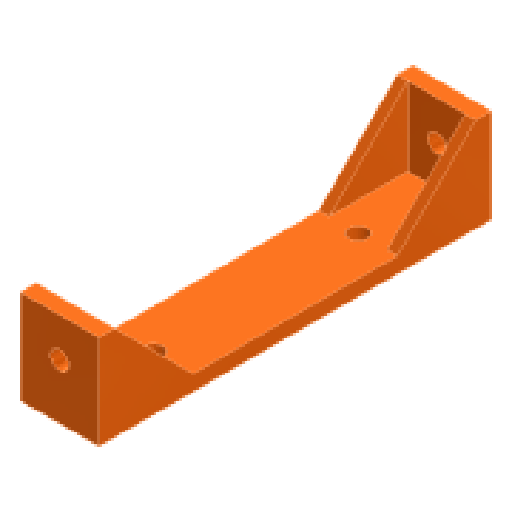
# Autodesk Inventor part: Frame_Brace_Mount
Saved by Autodesk Inventor 2023.2 (Build 272271000, 271)
## iProperties
Created: 2023-02-02
Part Number: Frame_Brace_Mount
Material: ABS Plastic
Document SubType Name: Modeling
Designer: remop
Density: 1.06 g/cm^3
Appearance: Smooth - Light Orange
Author: remop
Autodesk Inventor part; units mm, degrees
ref_plane "YZ Plane" through (0, 0, 0) normal (1, 0, 0) x (0, 1, 0)
ref_plane "XZ Plane" through (0, 0, 0) normal (0, 1, 0) x (-1, 0, 0)
ref_plane "XY Plane" through (0, 0, 0) normal (0, 0, 1) x (1, 0, 0)
sketch "Sketch1" plane through (0, 0, 0) normal (0, 1, 0) x (-1, 0, 0)
  line L0 (-7.5, 37.5) -> (7.5, 37.5)
  line L1 (7.5, 37.5) -> (7.5, -37.5)
  line L2 (7.5, -37.5) -> (-7.5, -37.5)
  line L3 (-7.5, -37.5) -> (-7.5, 37.5)
  line L4 (-7.5, 37.5) -> (7.5, -37.5) construction
  line L5 (7.5, 37.5) -> (-7.5, -37.5) construction
  circle A0 centre (0, 19.5) radius 1.75
  circle A1 centre (0, -19.5) radius 1.75
  point P0 (0, 0)
  point P1 (0, -37.5)
  dimension "d0" = 15
  dimension "d1" = 75
  dimension "d13" = 18
  dimension "d14" = 18
  dimension "d16" = 3.5
  constraints: 12 end point, 3 midpoint, 2 centre point, 2 parallel, 2 vertical alignment, 1 equal radius, 1 horizontal, 1 perpendicular
  measures "d0" distance of L1.end L2.end
  measures "d1" distance of L2.end L0.start
  measures "d13" distance from line of L0 A0.centre
  measures "d14" distance from line of L2 A1.centre
  measures "d16" diameter of A1
extrude "Extrusion1" add sketch "Sketch1" along normal blind 3
sketch "Sketch2" plane through (-7.5, 0, 37.5) normal (0, 0, 1) x (1, 0, 0)
  line L0 (0, 0) -> (15, 0) projected
  line L1 (15, 0) -> (15, 3) projected
  line L2 (0, 3) -> (15, 3) projected
  line L3 (0, 0) -> (0, 3) projected
  line L4 (15, 3) -> (0, 3) projected
  line L5 (0, 3) -> (15, 3)
  line L6 (15, 3) -> (15, 18)
  line L7 (15, 18) -> (0, 18)
  line L8 (0, 18) -> (0, 3)
  circle A0 centre (7.5, 10.5) radius 1.75
  point P0 (7.5, 0)
  point P1 (7.5, 18)
  point P2 (0, 10.5)
  dimension "d15" = 3.5
  constraints: 8 end point, 2 midpoint, 2 parallel, 2 perpendicular, 1 centre point, 1 coincident, 1 horizontal, 1 horizontal alignment, 1 vertical alignment
  measures "d15" diameter of A0
extrude "Extrusion2" add sketch "Sketch2" against normal blind 3 contours L8 L7 L6 L2
sketch "Sketch3" plane through (7.5, 0, -37.5) normal (0, 0, -1) x (-1, 0, 0)
  line L0 (15, 18) -> (0, 18) projected
  line L1 (0, 18) -> (0, 3) projected
  line L2 (15, 3) -> (0, 3) projected
  line L3 (15, 3) -> (15, 18) projected
  circle A0 centre (7.5, 10.5) radius 1.75 projected
  point P0 (7.5, 0)
extrude "Extrusion3" add sketch "Sketch3" against normal blind 3
sketch "Sketch4" plane through (7.5, 0, 37.5) normal (1, 0, 0) x (0, 0, -1)
  line L0 (0, 0) -> (75, 0) projected
  line L1 (75, 0) -> (75, 18) projected
  line L2 (75, 18) -> (72, 18) projected
  line L3 (72, 3) -> (72, 18) projected
  line L4 (3, 3) -> (72, 3) projected
  line L5 (3, 18) -> (3, 3) projected
  line L6 (0, 18) -> (3, 18) projected
  line L7 (0, 0) -> (0, 18) projected
  line L8 (3, 18) -> (18, 3)
  line L9 (72, 3) -> (72, 18) projected
  line L10 (72, 18) -> (57, 3)
  line L11 (72, 3) -> (3, 3) projected
  point P0 (37.5, 0)
  dimension "d8" = 45
  constraints: 4 end point, 2 point on line, 1 perpendicular
  measures "d8" angle of L4 L8
extrude "Extrusion4" add sketch "Sketch4" against normal blind 2 contours L8 L4 L5 | L3 L4 L10
sketch "Sketch5" plane through (-7.5, 0, -37.5) normal (-1, 0, 0) x (0, 0, 1)
  line L0 (18, 3) -> (3, 3) projected
  line L1 (18, 3) -> (3, 18) projected
  line L2 (3, 3) -> (3, 18) projected
  line L3 (72, 3) -> (57, 3) projected
  line L4 (72, 18) -> (72, 3) projected
  line L5 (72, 18) -> (57, 3) projected
  point P0 (37.5, 0)
extrude "Extrusion5" add sketch "Sketch5" against normal blind 2
equation "\"d14\" = d13"
body "Solid1"
